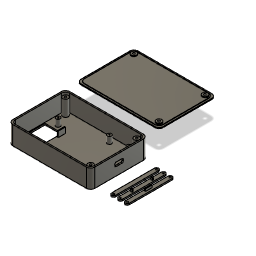
outdoor sensor v5 (Autodesk Fusion 360 design; units mm, degrees)
Autodesk Fusion 360 part; units mm, degrees
note: some values were not read from the file. Set by a fixed rule: which sketch regions a step uses.
sketch "Sketch1" plane through (0, 0, 0) normal (0, 1, 0) x (1, 0, 0)
  line L0 (-40, 25) -> (32, 25)
  line L1 (32, 25) -> (32, -25)
  line L2 (32, -25) -> (-40, -25)
  line L3 (-40, -25) -> (-40, 25)
  constraint horizontal L0
  constraint vertical L1
  constraint horizontal L2
  constraint vertical L3
extrude "Extrude1" add sketch "Sketch1" along normal blind 1.2 makes body 1
sketch "Sketch2" plane through (0, 1.2, 0) normal (0, 1, 0) x (-1, 0, 0)
  line L0 (40, 25) -> (-32, 25)
  line L1 (-32, 25) -> (-32, -25)
  line L2 (-32, -25) -> (40, -25)
  line L3 (40, -25) -> (40, 25)
  line L4 (38.8, -23.8) -> (-30.8, -23.8)
  line L5 (-30.8, -23.8) -> (-30.8, 23.8)
  line L6 (-30.8, 23.8) -> (38.8, 23.8)
  line L7 (38.8, 23.8) -> (38.8, -23.8)
  constraint horizontal L4
  constraint vertical L5
  constraint horizontal L6
  constraint vertical L7
extrude "Extrude2" add sketch "Sketch2" along normal blind 40 bodies 1
sketch "Sketch3" plane through (0, 1.2, 0) normal (0, 1, 0) x (-1, 0, 0)
  line L0 (-30.8, 23.8) -> (-30.8, -23.8)
  line L1 (-30.8, -23.8) -> (38.8, -23.8)
  line L2 (38.8, -23.8) -> (38.8, 23.8)
  line L3 (38.8, 23.8) -> (-30.8, 23.8)
  line L4 (38, 15) -> (23, 15)
  line L5 (23, 15) -> (23, -5)
  line L6 (23, -5) -> (38, -5)
  line L7 (38, -5) -> (38, 15)
  constraint horizontal L4
  constraint vertical L5
  constraint horizontal L6
  constraint vertical L7
extrude "Extrude3" cut sketch "Sketch3" against normal blind 1.2 contours L4 L5 L6 L7 bodies 1
sketch "Sketch4" plane through (0, 1.2, 0) normal (0, 1, 0) x (-1, 0, 0)
  line L0 (23, 15) -> (38, 15)
  line L1 (38, 15) -> (38, -5)
  line L2 (38, -5) -> (23, -5)
  line L3 (23, -5) -> (23, 15)
  line L4 (-30.8, 23.8) -> (-30.8, -23.8)
  line L5 (-30.8, -23.8) -> (38.8, -23.8)
  line L6 (38.8, -23.8) -> (38.8, 23.8)
  line L7 (38.8, 23.8) -> (-30.8, 23.8)
  circle A0 centre (30.5, 17.25) radius 0.6
  circle A1 centre (30.5, 17.25) radius 1.8
  circle A2 centre (30.555, -9.025) radius 0.6
  circle A3 centre (30.555, -9.025) radius 1.8
  dimension "d15" = 1.2
  dimension "d16" = 3.6
  dimension "d17" = 1.2
  dimension "d18" = 3.6
  constraint concentric A0 A1
  constraint concentric A2 A3
  measures "d15" diameter of A0
  measures "d16" diameter of A1
  measures "d17" diameter of A2
  measures "d18" diameter of A3
extrude "Extrude4" add sketch "Sketch4" along normal blind 6 contours A1 | A3 bodies 1
sketch "Sketch5" plane through (0, 1.2, 0) normal (0, 1, 0) x (-1, 0, 0)
  circle A0 centre (30.5, 17.25) radius 1.8
  line L0 (23, 15) -> (38, 15)
  line L1 (38, 15) -> (38, -5)
  line L2 (38, -5) -> (23, -5)
  line L3 (23, -5) -> (23, 15)
  line L4 (-30.8, 23.8) -> (-30.8, -23.8)
  line L5 (-30.8, -23.8) -> (38.8, -23.8)
  line L6 (38.8, -23.8) -> (38.8, 23.8)
  line L7 (38.8, 23.8) -> (-30.8, 23.8)
  circle A1 centre (30.555, -9.025) radius 1.8
  line L8 (21.4, 0) -> (22.2, 0)
  line L9 (22.2, 0) -> (22.2, -6.4)
  line L10 (22.2, -6.4) -> (21.4, -6.4)
  line L11 (21.4, -6.4) -> (21.4, 0)
  constraint horizontal L8
  constraint vertical L9
  constraint horizontal L10
  constraint vertical L11
extrude "Extrude5" add sketch "Sketch5" along normal blind 3.4 contours L8 L9 L10 L11 bodies 1
sketch "Sketch6" plane through (0, 1.2, 0) normal (0, 1, 0) x (-1, 0, 0)
  line L0 (21.4, -6.4) -> (21.4, 0)
  line L1 (21.4, 0) -> (22.2, 0)
  line L2 (22.2, 0) -> (22.2, -6.4)
  line L3 (22.2, -6.4) -> (21.4, -6.4)
  circle A0 centre (30.5, 17.25) radius 1.8
  line L4 (23, 15) -> (38, 15)
  line L5 (38, 15) -> (38, -5)
  line L6 (38, -5) -> (23, -5)
  line L7 (23, -5) -> (23, 15)
  line L8 (-30.8, 23.8) -> (-30.8, -23.8)
  line L9 (-30.8, -23.8) -> (38.8, -23.8)
  line L10 (38.8, -23.8) -> (38.8, 23.8)
  line L11 (38.8, 23.8) -> (-30.8, 23.8)
  circle A1 centre (30.555, -9.025) radius 1.8
  circle A2 centre (-5, -18.55) radius 0.6
  circle A3 centre (-5, -18.55) radius 1.8
  circle A4 centre (-5, 19.05) radius 0.6
  circle A5 centre (-5, 19.05) radius 1.8
  dimension "d23" = 1.2
  dimension "d24" = 3.6
  dimension "d25" = 1.2
  dimension "d26" = 3.6
  constraint concentric A2 A3
  constraint concentric A4 A5
  measures "d23" diameter of A2
  measures "d24" diameter of A3
  measures "d25" diameter of A4
  measures "d26" diameter of A5
extrude "Extrude6" add sketch "Sketch6" along normal blind 6 contours A3 | A5 bodies 1
sketch "Sketch7" plane through (0, 0, 0) normal (0, 1, 0) x (1, 0, 0)
  line L0 (26.1999, 36.8) -> (26.1999, 36.7999)
  line L1 (24.3999, 38.6) -> (-13.2, 38.6)
  arc A0 (-13.2, 38.6) -> (-13.1777, 35.0001) centre (-13.2, 36.8) ccw
  arc A1 (26.1999, 36.7999) -> (24.3999, 38.6) centre (24.3999, 36.8) ccw
  line L2 (-13.1777, 35.0001) -> (24.3999, 35)
  arc A2 (24.3999, 35) -> (26.1999, 36.8) centre (24.3999, 36.8) ccw
  point P0 (-15, 35)
  point P1 (-15, 38.6)
  dimension "d30" = 1.8
  dimension "d32" = 1.8
  dimension "d33" = 1.8
  constraint horizontal L1
  constraint coincident P1 L1
  constraint tangent L1 A0
  constraint tangent L1 A1
  constraint tangent L0 A2
  constraint tangent L2 A2
  measures "d30" radius of A0
  measures "d32" radius of A1
  measures "d33" radius of A2
extrude "Extrude7" add sketch "Sketch7" along normal blind 1.2 separate body makes body 2
sketch "Sketch8" plane through (0, 1.2, 0) normal (0, 1, 0) x (-1, 0, 0)
  arc A0 (-24.3999, -35) -> (-24.3999, -38.6) centre (-24.3999, -36.8) ccw
  line L0 (-24.3999, -38.6) -> (13.2, -38.6)
  arc A1 (13.2, -38.6) -> (13.1777, -35.0001) centre (13.2, -36.8) ccw
  line L1 (13.1777, -35.0001) -> (-24.3999, -35)
  circle A2 centre (13.2, -36.8) radius 0.8
  circle A3 centre (-24.3999, -36.8) radius 0.8
  dimension "d36" = 1.6
  dimension "d37" = 1.6
  constraint concentric A1 A2
  constraint concentric A0 A3
  measures "d36" diameter of A2
  measures "d37" diameter of A3
extrude "Extrude8" cut sketch "Sketch8" against normal blind 1.2 contours A2 | A3 bodies 2
extrude "Extrude9" cut 1 faces at (-15.6, 41.2, -24.6) along direction (0, -1, 0) blind 10 on bodies 1 bodies 1
fillet "Fillet1" radius 3.6 8 edges at (-40, 15.6, 25) (32, 15.6, 25) (-40, 15.6, -25) (32, 15.6, -25) (-38.8, 16.2, -23.8) (30.8, 16.2, -23.8) (30.8, 16.2, 23.8) (-38.8, 16.2, 23.8) on bodies 1
sketch "Sketch10" plane through (0, 1.2, 0) normal (0, 1, 0) x (-1, 0, 0)
  circle A0 centre (13.2, -36.8) radius 0.8
  circle A1 centre (-24.3999, -36.8) radius 0.8
  arc A2 (-24.3999, -35) -> (-24.3999, -38.6) centre (-24.3999, -36.8) ccw
  line L0 (-24.3999, -38.6) -> (13.2, -38.6)
  arc A3 (13.2, -38.6) -> (13.1777, -35.0001) centre (13.2, -36.8) ccw
  line L1 (13.1777, -35.0001) -> (-24.3999, -35)
  line L2 (-2.6, -36.8) -> (-8.6, -36.8)
  line L3 (-8.6, -36.8) -> (-8.6, -37.6)
  line L4 (-8.6, -37.6) -> (-2.6, -37.6)
  line L5 (-2.6, -37.6) -> (-2.6, -36.8)
  dimension "d46" = 6
  dimension "d79" = 0.8
  constraint vertical L3
  constraint horizontal L4
  constraint vertical L5
  measures "d46" distance of L2.start L2.end
  measures "d79" distance of L2.start L4.end
extrude "Extrude10" add sketch "Sketch10" along normal blind 2 contours L2 L3 L4 L5 bodies 2
sketch "Sketch11" plane through (0, 1.2, 0) normal (0, 1, 0) x (-1, 0, 0)
  arc A0 (38.8, 20.2) -> (35.2, 23.8) centre (35.2, 20.2) ccw
  line L0 (35.2, 23.8) -> (-27.2, 23.8)
  arc A1 (-27.2, 23.8) -> (-30.8, 20.2) centre (-27.2, 20.2) ccw
  line L1 (-30.8, 20.2) -> (-30.8, -20.2)
  arc A2 (-30.8, -20.2) -> (-27.2, -23.8) centre (-27.2, -20.2) ccw
  line L2 (-27.2, -23.8) -> (35.2, -23.8)
  arc A3 (35.2, -23.8) -> (38.8, -20.2) centre (35.2, -20.2) ccw
  line L3 (38.8, -20.2) -> (38.8, 20.2)
  circle A4 centre (-5, -18.55) radius 1.8
  line L4 (21.4, -6.4) -> (21.4, 0)
  line L5 (21.4, 0) -> (22.2, 0)
  line L6 (22.2, 0) -> (22.2, -6.4)
  line L7 (22.2, -6.4) -> (21.4, -6.4)
  circle A5 centre (30.5, 17.25) radius 1.8
  line L8 (23, 15) -> (38, 15)
  line L9 (38, 15) -> (38, -5)
  line L10 (38, -5) -> (23, -5)
  line L11 (23, -5) -> (23, 15)
  circle A6 centre (30.555, -9.025) radius 1.8
  circle A7 centre (-5, 19.05) radius 1.8
  circle A8 centre (-21.9978, -18.55) radius 0.6
  circle A9 centre (-21.9978, -18.55) radius 1.8
  circle A10 centre (-21.9978, 19.05) radius 0.6
  circle A11 centre (-21.9978, 19.05) radius 1.8
  dimension "d49" = 1.2
  dimension "d50" = 3.6
  dimension "d51" = 1.2
  dimension "d52" = 3.6
  constraint concentric A8 A9
  constraint concentric A10 A11
  measures "d49" diameter of A8
  measures "d50" diameter of A9
  measures "d51" diameter of A10
  measures "d52" diameter of A11
extrude "Extrude11" add sketch "Sketch11" along normal blind 6 contours A9 | A11 bodies 1
extrude "Extrude12" add 1 faces at (-21.6667, 4.6, -2.1333) along direction (0, 1, 0) blind 1.5 on bodies 1 bodies 1
move_face "MoveFace1" by (3.3561, 0, -8.6955) 1 faces at (6.6074, 1.2, -35.6001) on bodies 2
sketch "Sketch12" plane through (0, 0, 0) normal (0, 1, 0) x (1, 0, 0)
  arc A0 (-13.2, 44.6) -> (-13.1777, 41.0001) centre (-13.2, 42.8) ccw
  line L0 (-13.1777, 41.0001) -> (24.3999, 41)
  line L1 (24.3999, 44.6) -> (-13.2, 44.6)
  arc A1 (26.1999, 42.7999) -> (24.3999, 44.6) centre (24.3999, 42.8) ccw
  arc A2 (24.3999, 41) -> (26.1999, 42.8) centre (24.3999, 42.8) ccw
  circle A3 centre (-24.3999, -30.8) radius 0.8
  circle A4 centre (13.2, -30.8) radius 0.8
  arc A5 (-13.2, 38.6) -> (-13.1777, 35.0001) centre (-13.2, 36.8) ccw
  line L2 (-13.1777, 35.0001) -> (24.3999, 35)
  line L3 (24.3999, 38.6) -> (-13.2, 38.6)
  arc A6 (26.1999, 36.7999) -> (24.3999, 38.6) centre (24.3999, 36.8) ccw
  arc A7 (24.3999, 35) -> (26.1999, 36.8) centre (24.3999, 36.8) ccw
  circle A8 centre (-24.3999, -36.8) radius 0.8
  circle A9 centre (13.2, -36.8) radius 0.8
  arc A10 (-13.2, 50.6) -> (-13.1777, 47.0001) centre (-13.2, 48.8) ccw
  line L4 (-13.1777, 47.0001) -> (24.3999, 47)
  line L5 (24.3999, 50.6) -> (-13.2, 50.6)
  arc A11 (26.1999, 48.7999) -> (24.3999, 50.6) centre (24.3999, 48.8) ccw
  arc A12 (24.3999, 47) -> (26.1999, 48.8) centre (24.3999, 48.8) ccw
  circle A13 centre (-24.3999, -24.8) radius 0.8
  circle A14 centre (13.2, -24.8) radius 0.8
  circle A15 centre (-13.2, 48.8) radius 0.8
  circle A16 centre (24.3999, 48.8) radius 0.8
  circle A17 centre (-13.2, 42.8) radius 0.6
  circle A18 centre (24.3999, 42.8) radius 0.6
  dimension "d57" = 1.8
  dimension "d58" = 1.8
  dimension "d59" = 1.8
  dimension "d60" = 1.8
  dimension "d61" = 1.8
  dimension "d62" = 1.8
  dimension "d63" = 1.8
  dimension "d64" = 1.8
  dimension "d65" = 1.8
  dimension "d68" = 1.6
  dimension "d69" = 1.6
  dimension "d70" = 1.2
  dimension "d71" = 1.2
  constraint horizontal L1
  constraint tangent A0 L1
  constraint tangent L1 A1
  constraint tangent L0 A2
  constraint horizontal L3
  constraint tangent A5 L3
  constraint tangent L3 A6
  constraint tangent L2 A7
  constraint horizontal L5
  constraint tangent A10 L5
  constraint tangent L5 A11
  constraint tangent L4 A12
  constraint concentric A10 A15
  constraint concentric A12 A16
  constraint concentric A0 A17
  constraint concentric A2 A18
  measures "d57" radius of A0
  measures "d58" radius of A1
  measures "d59" radius of A2
  measures "d60" radius of A5
  measures "d61" radius of A6
  measures "d62" radius of A7
  measures "d63" radius of A10
  measures "d64" radius of A11
  measures "d65" radius of A12
  measures "d68" diameter of A15
  measures "d69" diameter of A16
  measures "d70" diameter of A17
  measures "d71" diameter of A18
extrude "Extrude13" add sketch "Sketch12" along normal blind 1.2 separate body contours A0 L0 L1 A1 A2 | A10 L4 L5 A11 A12 makes body 3 at (11.6264, 0, -50.1157) makes body 4 at (-0.6592, 0, -42.0821)
sketch "Sketch13" plane through (0, 1.2, 0) normal (0, 1, 0) x (-1, 0, 0)
  circle A0 centre (-24.3999, -42.8) radius 0.6
  circle A1 centre (13.2, -42.8) radius 0.6
  arc A2 (-24.3999, -41) -> (-24.3999, -44.6) centre (-24.3999, -42.8) ccw
  line L0 (-24.3999, -44.6) -> (13.2, -44.6)
  arc A3 (13.2, -44.6) -> (13.1777, -41.0001) centre (13.2, -42.8) ccw
  line L1 (13.1777, -41.0001) -> (-24.3999, -41)
  line L2 (2.95, -43.6) -> (3.75, -43.6)
  line L3 (3.75, -43.6) -> (3.75, -42)
  line L4 (3.75, -42) -> (2.95, -42)
  line L5 (2.95, -42) -> (2.95, -43.6)
  line L6 (-14.15, -43.6) -> (-14.95, -43.6)
  line L7 (-14.95, -43.6) -> (-14.95, -42)
  line L8 (-14.95, -42) -> (-14.15, -42)
  line L9 (-14.15, -42) -> (-14.15, -43.6)
  constraint horizontal L2
  constraint vertical L3
  constraint horizontal L4
  constraint vertical L5
  constraint horizontal L6
  constraint vertical L7
  constraint horizontal L8
  constraint vertical L9
extrude "Extrude14" add sketch "Sketch13" along normal blind 2 contours L2 L3 L4 L5 | L6 L7 L8 L9 bodies 4
sketch "Sketch14" plane through (0, 1.2, 0) normal (0, 1, 0) x (-1, 0, 0)
  circle A0 centre (-21.9978, -18.55) radius 1.8
  arc A1 (38.8, 20.2) -> (35.2, 23.8) centre (35.2, 20.2) ccw
  line L0 (35.2, 23.8) -> (-27.2, 23.8)
  arc A2 (-27.2, 23.8) -> (-30.8, 20.2) centre (-27.2, 20.2) ccw
  line L1 (-30.8, 20.2) -> (-30.8, -20.2)
  arc A3 (-30.8, -20.2) -> (-27.2, -23.8) centre (-27.2, -20.2) ccw
  line L2 (-27.2, -23.8) -> (35.2, -23.8)
  arc A4 (35.2, -23.8) -> (38.8, -20.2) centre (35.2, -20.2) ccw
  line L3 (38.8, -20.2) -> (38.8, 20.2)
  circle A5 centre (-5, -18.55) radius 1.8
  line L4 (21.4, -6.4) -> (21.4, 0)
  line L5 (21.4, 0) -> (22.2, 0)
  line L6 (22.2, 0) -> (22.2, -6.4)
  line L7 (22.2, -6.4) -> (21.4, -6.4)
  circle A6 centre (30.5, 17.25) radius 1.8
  line L8 (23, 15) -> (38, 15)
  line L9 (38, 15) -> (38, -5)
  line L10 (38, -5) -> (23, -5)
  line L11 (23, -5) -> (23, 15)
  circle A7 centre (30.555, -9.025) radius 1.8
  circle A8 centre (-5, 19.05) radius 1.8
  circle A9 centre (-21.9978, 19.05) radius 1.8
sketch "Sketch16" plane through (32, 0, 0) normal (1, 0, 0) x (0, 0, -1)
  line L0 (21.4, 0) -> (21.4, 31.2)
  line L1 (21.4, 31.2) -> (-21.4, 31.2)
  line L2 (-21.4, 31.2) -> (-21.4, 0)
  line L3 (-21.4, 0) -> (21.4, 0)
  line L4 (2.7, 7.2) -> (-2.7, 7.2)
  line L5 (-3.7, 8.2) -> (-3.7, 9.6)
  line L6 (-2.7, 10.6) -> (2.7, 10.6)
  line L7 (3.7, 9.6) -> (3.7, 8.2)
  arc A0 (-2.7, 10.6) -> (-3.7, 9.6) centre (-2.7, 9.6) ccw
  arc A1 (3.7, 9.6) -> (2.7, 10.6) centre (2.7, 9.6) ccw
  arc A2 (2.7, 7.2) -> (3.7, 8.2) centre (2.7, 8.2) ccw
  arc A3 (-3.7, 8.2) -> (-2.7, 7.2) centre (-2.7, 8.2) ccw
  dimension "d91" = 1
  constraint horizontal L4
  constraint vertical L5
  constraint horizontal L6
  constraint vertical L7
  constraint tangent L5 A0
  constraint tangent L6 A0
  constraint tangent L6 A1
  constraint tangent L7 A1
  constraint equal A0 A1
  constraint tangent L4 A2
  constraint tangent L7 A2
  constraint equal A0 A2
  constraint tangent L4 A3
  constraint tangent L5 A3
  constraint equal A0 A3
  measures "d91" radius of A0
extrude "Extrude17" cut sketch "Sketch16" against normal blind 1.2 contours L4 L5 L6 L7 A0 A1 A2 A3 bodies 1
extrude "Extrude18" cut 1 faces at (-14.4, 31.2, -24.6) along direction (0, -1, 0) blind 5 on bodies 1 bodies 1
extrude "Extrude19" cut 1 faces at (-14.4, 26.2, -24.6) along direction (0, -1, 0) blind 5 on bodies 1 bodies 1
sketch "Sketch17" plane through (0, 1.2, 0) normal (0, 1, 0) x (-1, 0, 0)
  circle A0 centre (35.2, -20.2) radius 2.4
  circle A1 centre (-27.2, -20.2) radius 2.4
  circle A2 centre (-27.2, 20.2) radius 2.4
  circle A3 centre (35.2, -20.2) radius 1
  circle A4 centre (-27.2, -20.2) radius 1
  circle A5 centre (-27.2, 20.2) radius 1
  point P0 (35.2, -20.2)
  point P1 (-27.2, -20.2)
  point P2 (-27.2, 20.2)
  dimension "d98" = 4.8
  dimension "d99" = 4.8
  dimension "d100" = 4.8
  dimension "d101" = 2
  dimension "d102" = 2
  dimension "d103" = 2
  constraint coincident P0 A0.centre
  constraint coincident P1 A1.centre
  constraint coincident P2 A2.centre
  constraint concentric A0 A3
  constraint concentric A1 A4
  measures "d98" diameter of A0
  measures "d99" diameter of A1
  measures "d100" diameter of A2
  measures "d101" diameter of A3
  measures "d102" diameter of A4
  measures "d103" diameter of A5
extrude "Extrude20" cut 1 faces at (-14.4, 21.2, -24.6) along direction (0, -1, 0) blind 5 on bodies 1 bodies 1
extrude "Extrude21" add sketch "Sketch17" along normal blind 13.8 bodies 1
sketch "Sketch18" plane through (0, 16.2, 0) normal (0, 1, 0) x (-1, 0, 0)
  arc A0 (38.8, 20.2) -> (35.2, 23.8) centre (35.2, 20.2) ccw
  line L0 (38.8, 20.2) -> (38.8, -20.2)
  arc A1 (35.2, -23.8) -> (38.8, -20.2) centre (35.2, -20.2) ccw
  line L1 (35.2, -23.8) -> (-27.2, -23.8)
  arc A2 (-30.8, -20.2) -> (-27.2, -23.8) centre (-27.2, -20.2) ccw
  line L2 (-30.8, -20.2) -> (-30.8, 20.2)
  arc A3 (-27.2, 23.8) -> (-30.8, 20.2) centre (-27.2, 20.2) ccw
  line L3 (-27.2, 23.8) -> (35.2, 23.8)
  arc A4 (-32, -21.4) -> (-28.4, -25) centre (-28.4, -21.4) ccw
  line L4 (-28.4, -25) -> (36.4, -25)
  arc A5 (36.4, -25) -> (40, -21.4) centre (36.4, -21.4) ccw
  line L5 (40, -21.4) -> (40, 21.4)
  arc A6 (40, 21.4) -> (36.4, 25) centre (36.4, 21.4) ccw
  line L6 (36.4, 25) -> (-28.4, 25)
  arc A7 (-28.4, 25) -> (-32, 21.4) centre (-28.4, 21.4) ccw
  line L7 (-32, 21.4) -> (-32, -21.4)
  arc A8 (-35, 21.4) -> (-38.6, 25) centre (-38.6, 21.4) ccw
  line L8 (-36.4, 20) -> (-36.4, -20)
  line L9 (-35, -21.4) -> (-35, 21.4)
  line L10 (-38.6, 25) -> (-103.4, 25)
  line L11 (-102, 23.6) -> (-40, 23.6)
  arc A9 (-103.4, 25) -> (-107, 21.4) centre (-103.4, 21.4) ccw
  line L12 (-105.6, -20) -> (-105.6, 20)
  line L13 (-107, 21.4) -> (-107, -21.4)
  arc A10 (-107, -21.4) -> (-103.4, -25) centre (-103.4, -21.4) ccw
  line L14 (-103.4, -25) -> (-38.6, -25)
  line L15 (-40, -23.6) -> (-102, -23.6)
  arc A11 (-38.6, -25) -> (-35, -21.4) centre (-38.6, -21.4) ccw
  circle A12 centre (-39.8, -20.2) radius 2.4
  circle A13 centre (-39.8, -20.2) radius 1
  circle A14 centre (-102.2, -20.2) radius 1
  circle A15 centre (-102.2, -20.2) radius 2.4
  circle A16 centre (-102.2, 20.2) radius 2.4
  circle A17 centre (-102.2, 20.2) radius 1
  arc A18 (-40, -23.6) -> (-36.4, -20) centre (-40, -20) ccw
  arc A19 (-36.4, 20) -> (-40, 23.6) centre (-40, 20) ccw
  arc A20 (-102, 23.6) -> (-105.6, 20) centre (-102, 20) ccw
  arc A21 (-105.6, -20) -> (-102, -23.6) centre (-102, -20) ccw
  dimension "d110" = 3.6
  dimension "d111" = 3.6
  dimension "d112" = 3.6
  dimension "d113" = 3.6
  constraint tangent L15 A18
  constraint tangent L8 A18
  constraint tangent L11 A19
  constraint tangent L8 A19
  constraint tangent L11 A20
  constraint tangent L12 A20
  constraint tangent L12 A21
  constraint tangent L15 A21
  measures "d110" radius of A18
  measures "d111" radius of A19
  measures "d112" radius of A20
  measures "d113" radius of A21
extrude "Extrude22" add sketch "Sketch18" along normal blind 0.8 separate body contours A8 L9 L10 A9 L13 A10 L14 A11 makes body 5
extrude "Extrude23" add sketch "Sketch18" along normal blind 2 separate body contours A12 | A15 | A16 makes body 6 at (99.8119, 16.8667, 19.961) makes body 7 at (99.8119, 16.8667, -20.439) makes body 8 at (37.4119, 16.8667, -20.439)
extrude "Extrude24" add sketch "Sketch18" along normal blind 1.2 contours L8 L11 L12 L15 A18 A19 A20 A21 bodies 5 6 7 8
move_body "Move1" bodies 5 to x (1, 0, 0) y (0, 1, 0) z (0, 0, 1) at (-75, 0, -60)
move_body "Move2" bodies 4 3 2 to x (0, 0, -1) y (0, 1, 0) z (1, 0, 0) at (94.6, 0, 5.4)
